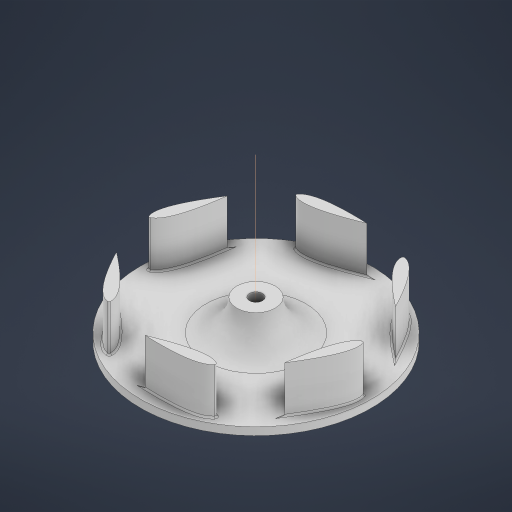
# Autodesk Inventor part: FanWing
Saved by Autodesk Inventor 2023 (Build 270158000, 158)
## iProperties
Created: 2023-02-14
Part Number: FanWing
Material: 一般
Document SubType Name: Modeling
Designer: neko2
Density: 1 g/cm^3
Appearance: 既定
Author: neko2
Autodesk Inventor part; units mm, degrees
ref_plane "YZ Plane" through (0, 0, 0) normal (1, 0, 0) x (0, 1, 0)
ref_plane "XZ Plane" through (0, 0, 0) normal (0, 1, 0) x (-1, 0, 0)
ref_plane "XY Plane" through (0, 0, 0) normal (0, 0, 1) x (1, 0, 0)
sketch "スケッチ1" plane through (0, 0, 0) normal (0, 1, 0) x (-1, 0, 0)
  circle A0 centre (0, 0) radius 7.5
  dimension "d0" = 15
  constraints: 1 centre point, 1 coincident
  measures "d0" diameter of A0
extrude "押し出し1" add sketch "スケッチ1" along normal blind 0.5
sketch "スケッチ2" plane through (0, 0.5, 0) normal (0, 1, 0) x (1, 0, 0)
  circle A0 centre (0, 0) radius 7.5 projected
  line L0 (-7, 0) -> (-5.6319, 3.7588)
  line L1 (-7, 0) -> (-7.5, 0.8) construction
  line L2 (-7.5, 0.8) -> (-5.6319, 3.7588) construction
  spline S0 degree 2 poles (-7, 0) (-7.5, 0.8) (-5.6319, 3.7588) knots 1 1 1 2 2 2
  line L3 (-7.5, 0) -> (-7.5, 3.2916)
  line L4 (-7, 0) -> (-6.1027, 0.2914) construction
  line L5 (-6.1027, 0.2914) -> (-5.6319, 3.7588) construction
  spline S1 degree 2 poles (-7, 0) (-6.1027, 0.2914) (-5.6319, 3.7588) knots 1 1 1 2 2 2
  dimension "d4" = 20
  dimension "d5" = 0.5
  dimension "d6" = 4
  dimension "d7" = 0.8
  constraints: 4 end point, 2 horizontal alignment, 2 vertical, 1 point on line, 1 symmetric about line, 7 other
  measures "d4" angle of L3 L0
  measures "d5" distance of L0.start L3.start
  measures "d6" distance of L0.start L0.end
  measures "d7" distance of L1.end L3.start
extrude "押し出し2" add sketch "スケッチ2" along normal blind 3 contours S0 L0 | L0 S1
fillet "フィレット1" radius 0.1 1 edges at (-7, 2, 0)
fillet "フィレット2" radius 0.1 3 edges at (-6.9877, 0.5, -0.0339) (-6.8705, 0.5, -1.4397) (-6.1738, 0.5, -1.1861)
pattern_circular "円形状パターン1" count 6 over 360 about axis through (0, 0, 0) along (0, 1, 0) of "押し出し2", "フィレット1", "フィレット2"
sketch "スケッチ3" plane through (0, 0.5, 0) normal (0, 1, 0) x (1, 0, 0)
  circle A0 centre (0, 0) radius 1.25
  dimension "d17" = 2.5
  constraints: 1 centre point, 1 coincident
  measures "d17" diameter of A0
extrude "押し出し3" add sketch "スケッチ3" along normal blind 2
fillet "フィレット3" radius 2 1 edges at (-1.25, 0.5, 0)
sketch "スケッチ4" plane through (0, 2.5, 0) normal (0, 1, 0) x (1, 0, 0)
  circle A0 centre (0, 0) radius 0.425
  dimension "d21" = 0.85
  constraints: 1 centre point, 1 coincident
  measures "d21" diameter of A0
extrude "押し出し4" cut sketch "スケッチ4" against normal through all
